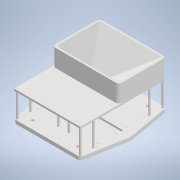
# Autodesk Inventor part: base_
Saved by Autodesk Inventor 2021 (Build 250183000, 183)
## iProperties
Created: 2021-11-22
Part Number: base_
Material: Generic
Document SubType Name: Modeling
Designer: techv
Density: 1 g/cm^3
Appearance: Default
Author: techv
Autodesk Inventor part; units mm, degrees
ref_plane "YZ Plane" through (0, 0, 0) normal (1, 0, 0) x (0, 1, 0)
sketch "Sketch1" plane through (0, 0, 0) normal (0, 1, 0) x (-1, 0, 0)
  line L0 (-65, 100) -> (65, 100) construction
  line L1 (65, 100) -> (65, -100) construction
  line L2 (65, -100) -> (-65, -100) construction
  line L3 (-65, -100) -> (-65, 100) construction
  line L4 (-65, 100) -> (65, -100) construction
  line L5 (65, 100) -> (-65, -100) construction
  line L6 (45, 110) -> (85, 110) construction
  line L7 (85, 110) -> (85, 90)
  line L8 (85, 90) -> (45, 90) construction
  line L9 (45, 90) -> (45, 110) construction
  line L10 (45, 110) -> (85, 90) construction
  line L11 (85, 110) -> (45, 90) construction
  line L12 (85, -90) -> (85, -110) construction
  line L13 (45, -90) -> (85, -90) construction
  line L14 (45, -110) -> (45, -90) construction
  line L15 (85, -110) -> (45, -110) construction
  line L16 (-45, 110) -> (-45, 90) construction
  line L17 (-85, 110) -> (-45, 110) construction
  line L18 (-85, 90) -> (-85, 110) construction
  line L19 (-45, 90) -> (-85, 90) construction
  line L20 (-45, -90) -> (-45, -110) construction
  line L21 (-85, -90) -> (-45, -90) construction
  line L22 (-85, -110) -> (-85, -90) construction
  line L23 (-45, -110) -> (-85, -110) construction
  line L24 (-95, -122.5) -> (95, -122.5)
  line L25 (95, -122.5) -> (95, 122.5)
  line L26 (95, 122.5) -> (-95, 122.5)
  line L27 (-95, 122.5) -> (-95, -122.5)
  line L28 (-95, -122.5) -> (95, 122.5) construction
  line L29 (95, -122.5) -> (-95, 122.5) construction
  line L30 (95, 122.5) -> (95, 72.5)
  line L31 (95, 72.5) -> (45, 72.5)
  line L32 (45, 72.5) -> (45, -72.5)
  line L33 (45, -72.5) -> (95, -72.5)
  line L34 (95, -72.5) -> (95, -122.5)
  line L35 (0, 122.5) -> (0, -122.5) construction
  line L36 (-65, 100) -> (-65, -100) construction
  line L37 (-95, -122.5) -> (-95, 122.5)
  line L38 (-95, 72.5) -> (-45, 72.5)
  line L39 (-45, 72.5) -> (-45, -72.5)
  line L40 (-45, -72.5) -> (-95, -72.5)
  line L41 (-95, -72.5) -> (-95, -122.5)
  circle A0 centre (-65, 100) radius 4
  circle A1 centre (-65, -100) radius 4
  circle A2 centre (65, 100) radius 4
  circle A3 centre (65, -100) radius 4
  line L42 (95, -122.5) -> (116.6001, 0)
  line L43 (95, -122.5) -> (219.3898, -122.5) construction
  line L44 (116.6001, 0) -> (95, 122.5)
  line L45 (-95, -122.5) -> (-116.6001, 0)
  line L46 (-116.6001, 0) -> (-95, 122.5)
  point P0 (0, 0)
  dimension "d0" = 130
  dimension "d1" = 200
  dimension "d2" = 40
  dimension "d3" = 20
  dimension "d6" = 200
  dimension "d9" = 130
  dimension "d12" = 190
  dimension "d13" = 245
  dimension "d14" = 50
  dimension "d15" = 50
  dimension "d16" = 90
  dimension "d17" = 145
  dimension "d18" = 90
  dimension "d19" = 8
  dimension "d22" = 200
  dimension "d25" = 130
  dimension "d125" = 80
  constraints: 94 end point, 8 midpoint, 7 parallel, 6 horizontal, 6 perpendicular, 5 symmetric about line, 4 centre point, 2 point on line, 2 vertical, 1 coincident, 1 equal length, 30 other
  measures "d0" distance of L1.end L2.end
  measures "d1" distance of L0.end L1.end
  measures "d2" distance of L7.end L8.end
  measures "d3" distance of L6.end L7.end
  measures "d6" distance of L6.end L12.start
  measures "d9" distance of L6.end L16.start
  measures "d12" distance of L26.end L25.end
  measures "d13" distance of L25.end L24.end
  measures "d14" distance of L25.end L30.end
  measures "d15" distance of L30.end L31.end
  measures "d16" angle of L30 L31
  measures "d17" distance of L31.end L32.end
  measures "d18" angle of L32 L31
  measures "d19" diameter of A0
  measures "d22" distance of A0.centre A1.centre
  measures "d25" distance of A0.centre A2.centre
  measures "d125" angle of L43 L42
extrude "Extrusion1" add sketch "Sketch1" along normal blind 10
ref_plane "Work Plane1" through (-81.8523, 27.75, -99.4789) normal (0, -1, 0) x (1, 0, 0)
sketch "Sketch5" plane through (0, 10, 0) normal (0, 1, 0) x (1, 0, 0)
  circle A0 centre (-25.5, 67.5) radius 1.5 projected
  circle A1 centre (-86.5, 67.5) radius 1.5 projected
  circle A2 centre (-25.5, 18.5) radius 1.5 projected
  circle A3 centre (-86.5, 18.5) radius 1.5 projected
  line L0 (-22, 71) -> (-22, 15) projected
  line L1 (-90, 71) -> (-22, 71) projected
  line L2 (-90, 15) -> (-90, 71) projected
  line L3 (-22, 15) -> (-90, 15) projected
  line L4 (-22, 15) -> (-90, 15) projected
  line L5 (-90, 15) -> (-90, 5) projected
  line L6 (-22, 5) -> (-90, 5) projected
  line L7 (-22, 15) -> (-22, 5) projected
  circle A4 centre (86.5, 67.5) radius 1.5 projected
  circle A5 centre (25.5, 67.5) radius 1.5 projected
  circle A6 centre (86.5, 18.5) radius 1.5 projected
  circle A7 centre (25.5, 18.5) radius 1.5 projected
  line L8 (90, 71) -> (90, 15) projected
  line L9 (22, 71) -> (90, 71) projected
  line L10 (22, 15) -> (22, 71) projected
  line L11 (90, 15) -> (22, 15) projected
  line L12 (90, 15) -> (22, 15) projected
  line L13 (22, 15) -> (22, 5) projected
  line L14 (90, 5) -> (22, 5) projected
  line L15 (90, 15) -> (90, 5) projected
  circle A8 centre (25.5, -62.5) radius 1.5 projected
  circle A9 centre (86.5, -62.5) radius 1.5 projected
  circle A10 centre (25.5, -13.5) radius 1.5 projected
  circle A11 centre (86.5, -13.5) radius 1.5 projected
  line L16 (22, -66) -> (22, -10) projected
  line L17 (90, -66) -> (22, -66) projected
  line L18 (90, -10) -> (90, -66) projected
  line L19 (22, -10) -> (90, -10) projected
  line L20 (22, -10) -> (90, -10) projected
  line L21 (90, -10) -> (90, 0) projected
  line L22 (22, 0) -> (90, 0) projected
  line L23 (22, -10) -> (22, 0) projected
  circle A12 centre (-86.5, -62.5) radius 1.5 projected
  circle A13 centre (-25.5, -62.5) radius 1.5 projected
  circle A14 centre (-86.5, -13.5) radius 1.5 projected
  circle A15 centre (-25.5, -13.5) radius 1.5 projected
  line L24 (-90, -66) -> (-90, -10) projected
  line L25 (-22, -66) -> (-90, -66) projected
  line L26 (-22, -10) -> (-22, -66) projected
  line L27 (-90, -10) -> (-22, -10) projected
  line L28 (-90, -10) -> (-22, -10) projected
  line L29 (-22, -10) -> (-22, 0) projected
  line L30 (-90, 0) -> (-22, 0) projected
  line L31 (-90, -10) -> (-90, 0) projected
  line L32 (-90, 5) -> (-22, 5)
  line L33 (-22, 5) -> (-22, 0)
  line L34 (-22, 0) -> (-90, 0)
  line L35 (-90, 0) -> (-90, 5)
  line L36 (22, 5) -> (90, 5)
  line L37 (90, 5) -> (90, 0)
  line L38 (90, 0) -> (22, 0)
  line L39 (22, 0) -> (22, 5)
  point P0 (0, 0)
  constraints: 16 end point, 4 parallel, 2 horizontal, 2 perpendicular
extrude "Extrusion5" cut sketch "Sketch5" against normal through all contours A0 | A1 | A2 | A3 | L33 L30 L35 L6 | A4 | A5 | A6 | A7 | L37 L22 L39 L14 | A8 | A9 | A10 | A11 | A12 | A13 | A14 | A15
sketch "Sketch6" plane through (0, 10, 0) normal (0, 1, 0) x (1, 0, 0)
  line L0 (12.5, -12.5) -> (-12.5, -12.5)
  line L1 (-12.5, -12.5) -> (-12.5, 12.5)
  line L2 (-12.5, 12.5) -> (12.5, 12.5)
  line L3 (12.5, 12.5) -> (12.5, -12.5)
  line L4 (12.5, -12.5) -> (-12.5, 12.5) construction
  line L5 (-12.5, -12.5) -> (12.5, 12.5) construction
  point P0 (0, 0)
  dimension "d51" = 25
  dimension "d52" = 25
  constraints: 12 end point, 2 midpoint, 2 parallel, 1 horizontal, 1 perpendicular
  measures "d51" distance of L1.end L2.end
  measures "d52" distance of L0.end L1.end
extrude "Extrusion6" cut sketch "Sketch6" against normal through all
fillet "Fillet3" radius 10 6 edges at (95, 5, 122.5) (116.6001, 5, 0) (95, 5, -122.5) (-95, 5, 122.5) (-116.6001, 5, 0) (-95, 5, -122.5)
ref_plane "Work Plane4" through (-81.8523, 35, -99.4789) normal (0, -1, 0) x (1, 0, 0)
sketch "Sketch2" plane through (0, 10, 0) normal (0, 1, 0) x (1, 0, 0)
  arc A0 (-80.6174, 104.2921) -> (-80.6174, 106.8579) centre (-78.775, 105.575) ccw
  arc A1 (-80.5189, 93.2107) -> (-80.5189, 95.6393) centre (-78.775, 94.425) ccw
  arc A2 (-29.1211, 106.7893) -> (-29.1211, 104.3607) centre (-30.865, 105.575) ccw
  arc A3 (-29.1211, 95.6393) -> (-29.1211, 93.2107) centre (-30.865, 94.425) ccw
  line L0 (-78.775, 94.425) -> (-30.865, 105.575) construction
  line L1 (-30.865, 94.425) -> (-78.775, 105.575) construction
  line L2 (-84.82, 115) -> (-24.82, 115) construction
  line L3 (-24.82, 115) -> (-24.82, 85) construction
  line L4 (-24.82, 85) -> (-84.82, 85) construction
  line L5 (-84.82, 85) -> (-84.82, 115) construction
  line L6 (-84.82, 115) -> (-24.82, 85) construction
  line L7 (-24.82, 115) -> (-84.82, 85) construction
  line L8 (-75.0118, 110) -> (-80.8, 110)
  arc A4 (-80.6174, 104.2921) -> (-80.642, 104.305) centre (-80.642, 104.275) ccw
  line L9 (-80.642, 104.305) -> (-81.85, 104.305)
  line L10 (-81.85, 104.305) -> (-81.85, 95.695)
  line L11 (-81.85, 95.695) -> (-80.6625, 95.695)
  arc A5 (-76.5, 94.425) -> (-80.6625, 95.695) centre (-78.775, 94.425) ccw
  arc A6 (-80.6625, 93.155) -> (-76.5, 94.425) centre (-78.775, 94.425) ccw
  line L12 (-80.6625, 93.155) -> (-81.85, 93.155)
  line L13 (-81.85, 93.155) -> (-81.85, 91.2)
  arc A7 (-81.85, 91.2) -> (-80.8, 90.15) centre (-80.8, 91.2) ccw
  line L14 (-80.8, 90.15) -> (-75.0119, 90.15)
  arc A8 (-75.12, 90.5) -> (-75.0118, 90.15) centre (-74.5, 90.5) ccw
  line L15 (-75.12, 90.5) -> (-75.12, 109.5)
  arc A9 (-75.0118, 109.85) -> (-75.12, 109.5) centre (-74.5, 109.5) ccw
  line L16 (-75.0118, 109.85) -> (-80.8, 109.85)
  arc A10 (-80.8, 109.85) -> (-81.85, 108.8) centre (-80.8, 108.8) ccw
  line L17 (-81.85, 108.8) -> (-81.85, 106.845)
  line L18 (-81.85, 106.845) -> (-80.642, 106.845)
  arc A11 (-80.642, 106.845) -> (-80.6174, 106.8579) centre (-80.642, 106.875) ccw
  arc A12 (-80.6174, 104.2921) -> (-80.6174, 106.8579) centre (-78.775, 105.575) ccw
  line L19 (-27.79, 106.845) -> (-27.79, 108.8)
  arc A13 (-27.79, 108.8) -> (-28.84, 109.85) centre (-28.84, 108.8) ccw
  line L20 (-28.84, 109.85) -> (-34.6281, 109.85)
  arc A14 (-34.52, 109.5) -> (-34.6282, 109.8499) centre (-35.14, 109.5) ccw
  line L21 (-34.52, 109.5) -> (-34.52, 90.5)
  arc A15 (-34.6282, 90.15) -> (-34.52, 90.5) centre (-35.14, 90.5) ccw
  line L22 (-34.6282, 90.15) -> (-28.84, 90.15)
  arc A16 (-28.84, 90.15) -> (-27.79, 91.2) centre (-28.84, 91.2) ccw
  line L23 (-27.79, 91.2) -> (-27.79, 93.155)
  line L24 (-27.79, 93.155) -> (-28.998, 93.155)
  arc A17 (-28.998, 93.155) -> (-29.0226, 93.1421) centre (-28.998, 93.125) ccw
  arc A18 (-29.0226, 95.7079) -> (-29.0226, 93.1421) centre (-30.865, 94.425) ccw
  arc A19 (-29.0226, 95.7079) -> (-28.998, 95.695) centre (-28.998, 95.725) ccw
  line L25 (-28.998, 95.695) -> (-27.79, 95.695)
  line L26 (-27.79, 95.695) -> (-27.79, 104.305)
  line L27 (-27.79, 104.305) -> (-28.998, 104.305)
  arc A20 (-28.998, 104.305) -> (-29.0226, 104.2921) centre (-28.998, 104.275) ccw
  arc A21 (-29.0226, 106.8579) -> (-29.0226, 104.2921) centre (-30.865, 105.575) ccw
  arc A22 (-29.0226, 106.8579) -> (-28.998, 106.845) centre (-28.998, 106.875) ccw
  line L28 (-28.998, 106.845) -> (-27.79, 106.845)
  line L29 (-84.82, 115) -> (-75.12, 115)
  line L30 (-75.12, 115) -> (-75.12, 85)
  line L31 (-75.12, 85) -> (-84.82, 85)
  line L32 (-84.82, 85) -> (-84.82, 115)
  line L33 (-24.82, 85) -> (-34.6282, 85)
  line L34 (-34.6282, 85) -> (-34.6282, 115)
  line L35 (-34.6282, 115) -> (-24.82, 115)
  line L36 (-24.82, 115) -> (-24.82, 85)
  point P0 (0, 0)
  point P1 (-54.82, 100)
extrude "Extrusion14" add sketch "Sketch2" along normal up to surface (25 mm away) contours A4 L9 L10 L11 A5 A6 L12 L13 A7 L14 L30 L31 L32 L29 L16 A10 L17 L18 A11 A0 | A0 A11 L18 L17 A10 L16 L30 L15 L14 A7 L13 L12 A6 A5 L11 L10 L9 A4 | L28 A22 A21 A20 L27 L26 L25 A19 A18 A17 L24 L23 A16 L22 A15 L21 A14 L20 A13 L19 | L19 A13 L20 L34 L35 L36 L33 L22 A16 L23 L24 A17 A18 A19 L25 L26 L27 A20 A21 A22 L28 | A14 L21 A15 L34
sketch "Sketch15" plane through (-34.6282, 35, -85) normal (0, 1, 0) x (1, 0, 0)
  arc A0 (5.5071, 21.7893) -> (5.5071, 19.3607) centre (3.7632, 20.575) ccw projected
  arc A1 (5.5071, 10.6393) -> (5.5071, 8.2107) centre (3.7632, 9.425) ccw projected
  arc A2 (-45.8906, 19.3607) -> (-45.8906, 21.7893) centre (-44.1468, 20.575) ccw projected
  arc A3 (-45.8906, 8.2107) -> (-45.8906, 10.6393) centre (-44.1468, 9.425) ccw projected
  circle A4 centre (-44.1468, 20.575) radius 2.125
  circle A5 centre (-44.1468, 9.425) radius 2.125
  circle A6 centre (3.7632, 20.575) radius 2.125
  circle A7 centre (3.7632, 9.425) radius 2.125
  point P0 (34.6282, -85)
  point P1 (-45.8906, 10.6393)
  point P2 (-45.8906, 8.2107)
  point P3 (-45.8906, 21.7893)
  point P4 (-45.8906, 19.3607)
  point P5 (5.5071, 10.6393)
  point P6 (5.5071, 21.7893)
  constraints: 4 coincident, 2 centre point, 2 concentric, 6 other
extrude "Extrusion15" cut sketch "Sketch15" against normal blind 15
pattern_linear "Rectangular Pattern7" count 2 spacing 110 along (1, 0, 0) of "Extrusion14", "Extrusion15"
sketch "Sketch16" plane through (0, 10, 0) normal (0, 1, 0) x (1, 0, 0)
  line L0 (95, 80) -> (-95, 80) construction
  line L1 (-95, 80) -> (-95, -80) construction
  line L2 (-95, -80) -> (95, -80) construction
  line L3 (95, -80) -> (95, 80) construction
  line L4 (95, 80) -> (-95, -80) construction
  line L5 (-95, 80) -> (95, -80) construction
  line L6 (-95, 80) -> (-15, 80) construction
  line L7 (-15, 80) -> (-15, -95) construction
  line L8 (-15, -95) -> (-95, -95) construction
  line L9 (-95, -95) -> (-95, 80) construction
  line L10 (95, 80) -> (15, 80) construction
  line L11 (15, 80) -> (15, -80) construction
  line L12 (15, -80) -> (95, -80) construction
  line L13 (95, -80) -> (95, 80) construction
  line L14 (-84.82, 115) -> (-84.82, 85) construction
  circle A0 centre (-78.775, 105.575) radius 2.125 construction
  circle A1 centre (-78.775, 94.425) radius 2.125 construction
  line L15 (-84.82, 85) -> (-75.12, 85) construction
  line L16 (-75.12, 85) -> (-75.12, 115) construction
  line L17 (-75.12, 115) -> (-84.82, 115) construction
  line L18 (-84.82, 115) -> (-84.82, 85) construction
  circle A2 centre (15, 80) radius 5
  circle A3 centre (95, 80) radius 5
  circle A4 centre (95, -80) radius 5
  circle A5 centre (15, -80) radius 5
  circle A6 centre (-95, -80) radius 5
  circle A7 centre (-15, -80) radius 5
  circle A8 centre (-15, 80) radius 5
  circle A9 centre (-95, 80) radius 5
  point P0 (0, 0)
  dimension "d137" = 190
  dimension "d138" = 160
  dimension "d139" = 80
  dimension "d140" = 175
  dimension "d141" = 80
  dimension "d142" = 10
  dimension "d143" = 10
  dimension "d144" = 10
  dimension "d145" = 10
  dimension "d146" = 10
  dimension "d147" = 10
  dimension "d148" = 10
  dimension "d149" = 10
  constraints: 26 end point, 8 centre point, 7 coincident, 5 parallel, 3 horizontal, 3 point on line, 2 midpoint, 2 perpendicular, 1 vertical, 3 other
  measures "d137" distance of L2.end L1.end
  measures "d138" distance of L1.end L1.start
  measures "d139" distance of L7.end L8.end
  measures "d140" distance of L6.end L7.end
  measures "d141" distance of L12.end L11.end
  measures "d142" diameter of A2
  measures "d143" diameter of A3
  measures "d144" diameter of A4
  measures "d145" diameter of A5
  measures "d146" diameter of A6
  measures "d147" diameter of A7
  measures "d148" diameter of A8
  measures "d149" diameter of A9
extrude "Extrusion16" add sketch "Sketch16" along normal blind 30
sketch "Sketch17" plane through (-95, 40, -80) normal (0, 1, 0) x (1, 0, 0)
  circle A0 centre (0, 0) radius 5 projected
  circle A1 centre (190, 0) radius 5 projected
  circle A2 centre (190, -160) radius 5 projected
  circle A3 centre (110, -160) radius 5 projected
  circle A4 centre (0, -160) radius 5 projected
  circle A5 centre (80, -160) radius 5 projected
  circle A6 centre (80, 0) radius 5 projected
  circle A7 centre (110, 0) radius 5 projected
  line L0 (0, 0) -> (80, -160) construction
  line L1 (80, 0) -> (0, -160) construction
  line L2 (190, -160) -> (110, 0) construction
  line L3 (190, 0) -> (110, -160) construction
  line L4 (-10, -167.5) -> (90, -167.5)
  line L5 (90, -167.5) -> (90, 7.5)
  line L6 (90, 7.5) -> (-10, 7.5)
  line L7 (-10, 7.5) -> (-10, -167.5)
  line L8 (-10, -167.5) -> (90, 7.5) construction
  line L9 (90, -167.5) -> (-10, 7.5) construction
  line L10 (100, -167.5) -> (200, -167.5)
  line L11 (200, -167.5) -> (200, 7.5)
  line L12 (200, 7.5) -> (100, 7.5)
  line L13 (100, 7.5) -> (100, -167.5)
  line L14 (100, -167.5) -> (200, 7.5) construction
  line L15 (200, -167.5) -> (100, 7.5) construction
  point P0 (95, -80)
  point P1 (40, -80)
  point P2 (150, -80)
  dimension "d152" = 100
  dimension "d153" = 175
  dimension "d154" = 100
  dimension "d155" = 175
  constraints: 32 end point, 6 midpoint, 4 parallel, 2 horizontal, 2 perpendicular
  measures "d152" distance of L6.end L5.end
  measures "d153" distance of L5.end L4.end
  measures "d154" distance of L12.end L11.end
  measures "d155" distance of L11.end L10.end
extrude "Extrusion17" add sketch "Sketch17" along normal blind 3 contours A0 | A1 | A2 | A3 | A4 | A5 | A6 | A7 | L7 L6 L5 L4 | L13 L12 L11 L10
sketch "Sketch18" plane through (0, 10, 0) normal (0, 1, 0) x (1, 0, 0)
  line L0 (90, -115) -> (-90, -115)
  line L1 (-90, -115) -> (-90, 115)
  line L2 (-90, 115) -> (90, 115)
  line L3 (90, 115) -> (90, -115)
  line L4 (90, -115) -> (-90, 115) construction
  line L5 (-90, -115) -> (90, 115) construction
  circle A0 centre (-90, 115) radius 5
  circle A1 centre (90, 115) radius 5
  circle A2 centre (90, -115) radius 5
  circle A3 centre (-90, -115) radius 5
  line L6 (-84.82, 85) -> (-84.82, 115) projected
  line L7 (-84.82, 115) -> (-75.12, 115) projected
  point P0 (0, 0)
  dimension "d158" = 180
  dimension "d159" = 230
  dimension "d160" = 10
  dimension "d161" = 10
  dimension "d162" = 10
  dimension "d163" = 10
  constraints: 12 end point, 4 centre point, 3 coincident, 2 midpoint, 2 parallel, 1 horizontal, 1 perpendicular
  measures "d158" distance of L1.end L2.end
  measures "d159" distance of L0.end L1.end
  measures "d160" diameter of A0
  measures "d161" diameter of A1
  measures "d162" diameter of A2
  measures "d163" diameter of A3
extrude "Extrusion18" cut sketch "Sketch18" against normal through all contours A3 L1 L0 | L0 L1 A3 | A2 L3 L0 | L0 L3 A2 | A0 L2 L1 | L1 L2 A0 | A1 L2 L3 | L3 L2 A1
body "Solid1"
